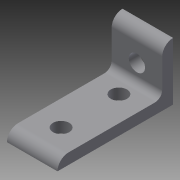
# Autodesk Inventor part: 4176
Saved by Autodesk Inventor 2014 SP2 (Build 180246200, 246)
## iProperties
Created: 2019-11-07
Part Number: 4176
Material: Generic
Catalog Web Link: www.cadenas.de
Description: 4176, 4376, 4176-Black, 4376-Black-Joining Plates - 3 Hole Inside Corner Bracket
Vendor: 8020
Document SubType Name: Modeling
Designer: psadmin
Manufacturer: 8020
Mass: 6.83763 g
Surface Area: 40.1375 cm^2
Volume: 6.83763 cm^3
Density: 1 g/cm^3
Appearance: PSOLRGB-191-191-191
Category: PARTsolutions
Company: 8020
Title: 4176
Author: Cadenas PARTsolutions
Comments: Joining Plates - 3 Hole Inside Corner Bracket
PSOL_IDENT_0: {$CADENAS_DATA\23d-libs\8020\inch\joining_plates\4176.prj},176 {VTYP=3D},{NB=4176},{LINA=4176},{NN=4
PSOL_IDENT_1: 176, 4376, 4176-Black, 4376-Black},{DATE=01.10.2019 06:04:23},{GEOMDATE=28.06.2017 15:47:04},{VERSIO
PSOL_IDENT_2: N=},{LINEID=10},{WBVAR=},{WBNUMERIC=}  {NB=4176},{LINA=4176},{KT=DUMMY},{PN=4176},{A=0.875},{B=2.000
PSOL_IDENT_3: },{C=1.000},{D=0.188},{E=0.281},{W=.040},{A1=0.500},{A2=1.500},{R=0.125},{COLOR=.75,.75,.75}
NN: 4176, 4376, 4176-Black, 4376-Black
NT: Joining Plates - 3 Hole Inside Corner Bracket
NB: 4176
NBSYN: $PN.
LINA: 4176
PN: 4176
A: 0.875
B: 2
C: 1
W: .040
SUPPLIER: 8020
ARTICLENO: 4176
BOMINFO: 4176
CREATOR: CADENAS GmbH
Autodesk Inventor part; units mm, degrees
ref_plane "YZ Plane" through (0, 0, 0) normal (1, 0, 0) x (0, 1, 0)
ref_plane "XZ Plane" through (0, 0, 0) normal (0, 1, 0) x (-1, 0, 0)
ref_plane "XY Plane" through (0, 0, 0) normal (0, 0, 1) x (1, 0, 0)
sketch "Sketch_1" plane through (0, 0, 0) normal (1, 0, 0) x (0, 1, 0)
  line L0 (0, 50.8) -> (0, 0)
  line L1 (0, 0) -> (25.4, 0)
  arc A0 (25.4, 0) -> (20.6248, 4.7752) centre (20.6248, 0) ccw
  line L2 (20.6248, 4.7752) -> (7.9502, 4.7752)
  arc A1 (4.7752, 7.9502) -> (7.9502, 4.7752) centre (7.9502, 7.9502) ccw
  line L3 (4.7752, 7.9502) -> (4.7752, 46.0248)
  arc A2 (4.7752, 46.0248) -> (0, 50.8) centre (0, 46.0248) ccw
  constraints: 8 end point, 6 point on circle, 3 centre point
extrude "Extrusion1" add sketch "Sketch_1" along normal mid plane 22.225
sketch "Sketch2" plane through (11.1125, 25.4, 0) normal (0, 0, -1) x (-1, 0, 0)
  point P0 (11.1125, -12.7)
hole "Hole1" at (0, 12.7, 0) direction (0, 0, 1) diameter 7.1374 depth 4.7752
sketch "Sketch3" plane through (-11.1125, 0, 0) normal (0, -1, 0) x (1, 0, 0)
  point P0 (11.1125, 12.7)
hole "Hole2" at (0, 0, 12.7) direction (0, 1, 0) diameter 7.1374 depth 4.7752
sketch "Sketch4" plane through (-11.1125, 0, 0) normal (0, -1, 0) x (1, 0, 0)
  point P0 (11.1125, 38.1)
hole "Hole3" at (0, 0, 38.1) direction (0, 1, 0) diameter 7.1374 depth 4.7752
body "Solid1"
